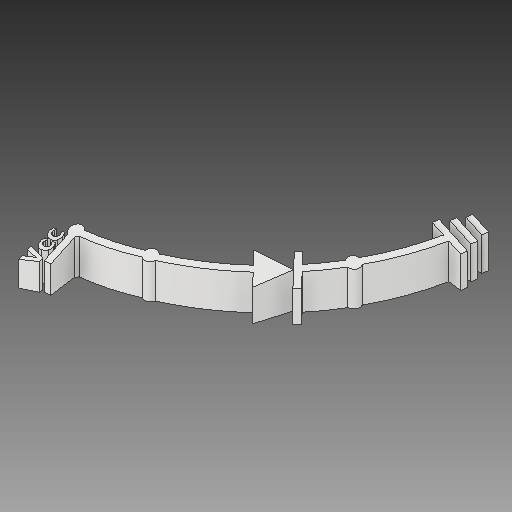
# Autodesk Inventor part: Mentor-Electrical text
Saved by Autodesk Inventor 2017 (Build 210142000, 142)
## iProperties
Created: 2016-02-20
Part Number: Mentor-Electrical text
Material: Generic
Document SubType Name: Modeling
Designer: RoksBot
Density: 1 g/cm^3
Appearance: White
Author: RoksBot
Autodesk Inventor part; units mm, degrees
ref_plane "YZ Plane" through (0, 0, 0) normal (1, 0, 0) x (0, 1, 0)
ref_plane "XZ Plane" through (0, 0, 0) normal (0, 1, 0) x (-1, 0, 0)
ref_plane "XY Plane" through (0, 0, 0) normal (0, 0, 1) x (1, 0, 0)
sketch "Sketch1" plane through (0, 0, 0) normal (0, 0, 1) x (1, 0, 0)
  line L0 (0, 0) -> (0, 8.6646) construction
  line L1 (20.9931, 1.27) -> (20.9931, 5.715)
  line L2 (20.9931, 5.715) -> (27.9781, 3.81)
  line L3 (27.9781, 3.81) -> (27.9781, 0)
  line L4 (27.9781, 0) -> (20.9931, 0)
  line L5 (20.9931, 1.27) -> (18.4531, 1.27)
  line L6 (18.4531, 1.27) -> (18.4531, 0)
  line L7 (18.4531, 0) -> (20.9931, 0)
  dimension "d0" = 20.9931
  dimension "d1" = 4.445
  dimension "d2" = 1.27
  dimension "d3" = 2.54
  dimension "d4" = 3.81
  dimension "d5" = 6.985
  constraints: 16 end point, 2 parallel, 2 perpendicular, 2 vertical, 1 horizontal, 1 horizontal alignment
  measures "d0" distance between parallel lines of L0 L1
  measures "d1" distance from line of L5 L1.end
  measures "d2" distance of L5.end L6.end
  measures "d3" distance between parallel lines of L1 L6
  measures "d4" distance of L2.end L3.end
  measures "d5" distance between parallel lines of L1 L3
revolve "Revolution1" add sketch "Sketch1" angle 360 about axis through (0, 0, 0) along (0, 1, 0)
sketch "Sketch2" plane through (0, 1.27, 0) normal (0, 1, 0) x (1, 0, 0)
  circle A0 centre (0, 0) radius 18.4531 projected
  circle A1 centre (0, 0) radius 20.9931 projected
  circle A2 centre (9.2057, -21.5899) radius 0.635
  arc A3 (9.6281, -21.1157) -> (15.5586, -17.2201) centre (0.0002, 0.0034) ccw
  arc A4 (9.8266, -21.7232) -> (15.9948, -17.6828) centre (0.0002, 0.0063) ccw
  line L0 (14.6057, -16.2094) -> (17.9425, -15.4197)
  line L1 (17.9425, -15.4197) -> (16.958, -18.7043)
  line L2 (16.958, -18.7043) -> (14.6057, -16.2094)
  line L3 (19.5807, -16.2316) -> (17.2284, -13.7366)
  line L4 (17.2284, -13.7366) -> (16.7663, -14.1722)
  line L5 (16.7663, -14.1722) -> (19.1186, -16.6672)
  line L6 (19.1186, -16.6672) -> (19.5807, -16.2316)
  line L7 (19.5807, -16.2316) -> (16.7663, -14.1722) construction
  line L8 (17.2284, -13.7366) -> (19.1186, -16.6672) construction
  arc A5 (18.0419, -14.5995) -> (19.8962, -11.96) centre (0.0423, 0.0164) ccw
  arc A6 (18.4961, -15.0813) -> (20.4645, -12.2797) centre (0.0089, 0.0003) ccw
  circle A7 centre (20.4475, -11.645) radius 0.635
  line L9 (22.5608, -1.3676) -> (24.4495, -1.6162)
  line L10 (24.4495, -1.6162) -> (24.3666, -2.2458)
  line L11 (24.3666, -2.2458) -> (22.4779, -1.9971)
  line L12 (22.4779, -1.9971) -> (22.5608, -1.3676)
  line L13 (22.5608, -1.3676) -> (24.3666, -2.2458) construction
  line L14 (24.4495, -1.6162) -> (22.4779, -1.9971) construction
  line L15 (22.0314, -3.2193) -> (24.5496, -3.5508)
  line L16 (24.5496, -3.5508) -> (24.6325, -2.9213)
  line L17 (24.6325, -2.9213) -> (22.1143, -2.5897)
  line L18 (22.1143, -2.5897) -> (22.0314, -3.2193)
  line L19 (22.0314, -3.2193) -> (24.6325, -2.9213) construction
  line L20 (24.5496, -3.5508) -> (22.1143, -2.5897) construction
  line L21 (21.3909, -4.4159) -> (24.7906, -4.8635)
  line L22 (24.7906, -4.8635) -> (24.8735, -4.2339)
  line L23 (24.8735, -4.2339) -> (21.4738, -3.7864)
  line L24 (21.4738, -3.7864) -> (21.3909, -4.4159)
  line L25 (21.3909, -4.4159) -> (24.8735, -4.2339) construction
  line L26 (24.7906, -4.8635) -> (21.4738, -3.7864) construction
  line L27 (0.0089, 0.0003) -> (33.281, -4.3801) construction
  arc A8 (20.9833, -11.3042) -> (23.3756, -4.6772) centre (0.0382, 0.0018) ccw
  arc A9 (20.3985, -11.0118) -> (22.7306, -4.5923) centre (0.0423, 0.0164) ccw
  line L28 (0.0423, 0.0164) -> (36.1387, 0.0164) construction
  circle A10 centre (0.0423, 0.0164) radius 23.4691 construction
  line L29 (0.0423, 0.0164) -> (5.4426, -41.0027) construction
  line L30 (0.0423, 0.0164) -> (0.0423, -40.9797) construction
  circle A11 centre (3.1056, -23.252) radius 0.635
  arc A12 (3.6155, -22.8735) -> (8.5745, -21.5207) centre (0.9957, -3.5037) ccw
  arc A13 (3.6826, -23.5172) -> (8.8414, -22.11) centre (1.5242, -5.4447) ccw
  line L31 (2.861, -23.8379) -> (3.2405, -26.7204)
  line L32 (3.2405, -26.7204) -> (3.87, -26.6375)
  line L33 (3.87, -26.6375) -> (3.4908, -23.7568)
  line L34 (1.3846, -26.2458) -> (2.9639, -26.5661)
  line L35 (2.9639, -26.5661) -> (3.016, -26.9616)
  line L36 (3.016, -26.9616) -> (1.5734, -27.6797)
  line L37 (1.5734, -27.6797) -> (1.5217, -27.2866)
  line L38 (1.5217, -27.2866) -> (2.5032, -26.8223)
  line L39 (2.5032, -26.8223) -> (1.4351, -26.6291)
  line L40 (1.4351, -26.6291) -> (1.3846, -26.2458)
  spline S0 degree 2 poles (2.8327, -25.3327) (2.8513, -25.4735) (2.811, -25.7167) (2.749, -25.8134) knots 0 0 0 1 2 2 2
  spline S1 degree 2 poles (2.749, -25.8134) (2.6854, -25.9077) (2.4739, -26.0327) (2.3221, -26.0527) knots 0 0 0 1 2 2 2
  spline S2 degree 2 poles (2.3221, -26.0527) (2.158, -26.0743) (1.9155, -26.0016) (1.8303, -25.9218) knots 0 0 0 1 2 2 2
  spline S3 degree 2 poles (1.8303, -25.9218) (1.7481, -25.8467) (1.6493, -25.6255) (1.6328, -25.5007) knots 0 0 0 1 2 2 2
  spline S4 degree 2 poles (1.6328, -25.5007) (1.6204, -25.4064) (1.6397, -25.212) (1.6748, -25.1102) knots 0 0 0 1 2 2 2
  line L41 (1.6748, -25.1102) -> (1.9785, -25.0702)
  line L42 (1.9785, -25.0702) -> (1.9845, -25.1155)
  spline S5 degree 2 poles (1.9845, -25.1155) (1.9666, -25.1403) (1.9256, -25.208) (1.9109, -25.2473) knots 0 0 0 1 2 2 2
  spline S6 degree 2 poles (1.9109, -25.2473) (1.894, -25.2894) (1.8774, -25.39) (1.8853, -25.45) knots 0 0 0 1 2 2 2
  spline S7 degree 2 poles (1.8853, -25.45) (1.9031, -25.5859) (2.1126, -25.7103) (2.2742, -25.689) knots 0 0 0 1 2 2 2
  spline S8 degree 2 poles (2.2742, -25.689) (2.4456, -25.6664) (2.5937, -25.485) (2.5763, -25.3528) knots 0 0 0 1 2 2 2
  spline S9 degree 2 poles (2.5763, -25.3528) (2.5674, -25.2854) (2.5236, -25.1891) (2.4967, -25.1552) knots 0 0 0 1 2 2 2
  spline S10 degree 2 poles (2.4967, -25.1552) (2.4712, -25.1225) (2.4179, -25.0772) (2.3971, -25.0612) knots 0 0 0 1 2 2 2
  line L43 (2.3971, -25.0612) -> (2.3911, -25.0159)
  line L44 (2.3911, -25.0159) -> (2.696, -24.9758)
  spline S11 degree 2 poles (2.696, -24.9758) (2.7135, -25.0046) (2.7583, -25.0797) (2.7748, -25.1199) knots 0 0 0 1 2 2 2
  spline S12 degree 2 poles (2.7748, -25.1199) (2.7963, -25.1694) (2.8229, -25.258) (2.8327, -25.3327) knots 0 0 0 1 2 2 2
  spline S13 degree 2 poles (2.6884, -24.2368) (2.707, -24.3777) (2.6667, -24.6209) (2.6047, -24.7175) knots 0 0 0 1 2 2 2
  spline S14 degree 2 poles (2.6047, -24.7175) (2.5412, -24.8118) (2.3297, -24.9368) (2.1778, -24.9568) knots 0 0 0 1 2 2 2
  spline S15 degree 2 poles (2.1778, -24.9568) (2.0138, -24.9784) (1.7712, -24.9057) (1.686, -24.826) knots 0 0 0 1 2 2 2
  spline S16 degree 2 poles (1.686, -24.826) (1.6039, -24.7508) (1.505, -24.5297) (1.4885, -24.4048) knots 0 0 0 1 2 2 2
  spline S17 degree 2 poles (1.4885, -24.4048) (1.4761, -24.3105) (1.4954, -24.1161) (1.5306, -24.0143) knots 0 0 0 1 2 2 2
  line L45 (1.5306, -24.0143) -> (1.8342, -23.9744)
  line L46 (1.8342, -23.9744) -> (1.8402, -24.0197)
  spline S18 degree 2 poles (1.8402, -24.0197) (1.8223, -24.0444) (1.7814, -24.1121) (1.7666, -24.1514) knots 0 0 0 1 2 2 2
  spline S19 degree 2 poles (1.7666, -24.1514) (1.7497, -24.1935) (1.7331, -24.2941) (1.741, -24.3541) knots 0 0 0 1 2 2 2
  spline S20 degree 2 poles (1.741, -24.3541) (1.7589, -24.49) (1.9683, -24.6144) (2.13, -24.5931) knots 0 0 0 1 2 2 2
  spline S21 degree 2 poles (2.13, -24.5931) (2.3014, -24.5706) (2.4494, -24.3891) (2.432, -24.2569) knots 0 0 0 1 2 2 2
  spline S22 degree 2 poles (2.432, -24.2569) (2.4231, -24.1896) (2.3793, -24.0932) (2.3524, -24.0594) knots 0 0 0 1 2 2 2
  spline S23 degree 2 poles (2.3524, -24.0594) (2.3269, -24.0266) (2.2736, -23.9813) (2.2528, -23.9653) knots 0 0 0 1 2 2 2
  line L47 (2.2528, -23.9653) -> (2.2469, -23.92)
  line L48 (2.2469, -23.92) -> (2.5518, -23.8799)
  spline S24 degree 2 poles (2.5518, -23.8799) (2.5693, -23.9087) (2.614, -23.9838) (2.6305, -24.024) knots 0 0 0 1 2 2 2
  spline S25 degree 2 poles (2.6305, -24.024) (2.652, -24.0735) (2.6786, -24.1622) (2.6884, -24.2368) knots 0 0 0 1 2 2 2
  point P0 (16.502, -16.7778)
  point P1 (15.7818, -17.4569)
  point P2 (18.1735, -15.2019)
  point P3 (23.4637, -1.8067)
  point P4 (23.332, -3.0703)
  point P5 (23.1322, -4.3249)
  point P6 (23.332, -3.0703)
  dimension "d48" = 1.27
  dimension "d50" = 0.635
  dimension "d52" = 7.62
  dimension "d53" = 3.429
  dimension "d54" = 0.635
  dimension "d55" = 3.429
  dimension "d56" = 1.27
  dimension "d57" = 0.635
  dimension "d59" = 3.81
  dimension "d60" = 3.429
  dimension "d61" = 2.54
  dimension "d62" = 1.905
  dimension "d63" = 0.635
  dimension "d64" = 0.635
  dimension "d65" = 0.635
  dimension "d67" = 0.635
  dimension "d74" = 7.5
  dimension "d75" = 0.3175
  dimension "d77" = 7.5
  dimension "d78" = 0.635
  constraints: 68 end point, 30 point on circle, 16 parallel, 12 centre point, 11 midpoint, 8 point on line, 5 perpendicular, 1 coincident, 1 concentric, 1 equal radius, 1 horizontal, 1 vertical, 8 other
  measures "d48" diameter of A2
  measures "d52" distance from line of L2 A2.centre
  measures "d53" distance of L1.end L0.start
  measures "d54" distance between parallel lines of L5 L3
  measures "d55" distance of L4.end L5.end
  measures "d56" diameter of A7
  measures "d59" distance of A5.start A7.centre
  measures "d60" distance of L21.start L21.end
  measures "d61" distance of L15.start L15.end
  measures "d62" distance of L10.end L11.end
  measures "d63" distance of L9.end L10.end
  measures "d64" distance between parallel lines of L23 L15
  measures "d65" distance between parallel lines of L17 L11
  measures "d74" angle of L28 L27
  measures "d75" radial gap between concentric circles of A9 A10
  measures "d77" angle of L30 L29
  measures "d78" distance of L31.end L32.end
extrude "Extrusion1" cut sketch "Sketch2" along normal through all contours A2 | A2 A3 L2 A4 | L5 L4 L3 L6 | A2 A13 A11 A12 | L2 L0 L1 | A11 | A11 L33 L32 L31 | A5 A7 A6 L3 | A7 | A9 L21 A8 A7 | L21 L24 L23 L22 | L9 L10 L11 L12 | L18 L17 L16 L15 | L34 L35 L36 L37 L38 L39 L40 | S0 S1 S2 S3 S4 L41 L42 S5 S6 S7 S8 S9 S10 L43 L44 S11 S12 | S13 S14 S15 S16 S17 L45 L46 S18 S19 S20 S21 S22 S23 L47 L48 S24 S25 keep common part
sketch "Sketch4" plane through (0, 1.27, 0) normal (0, 1, 0) x (1, 0, 0)
  line L0 (0, 0) -> (37.9646, 0)
  line L1 (37.9646, 0) -> (37.9646, -33.7381)
  line L2 (37.9646, -33.7381) -> (0, -33.7381)
  line L3 (0, -33.7381) -> (0, 0)
  constraints: 8 end point, 2 parallel, 1 horizontal, 1 perpendicular
extrude "Extrusion3" cut sketch "Sketch4" along normal through all both and the other way through all keep common part
equation "\"d48\" = d35"
equation "\"d52\" = d49"
equation "\"d53\" = d39"
equation "\"d54\" = d42"
equation "\"d55\" = d53"
equation "\"d56\" = d48"
equation "\"d59\" = d34"
equation "\"d65\" = d64"
equation "\"d26\" = d18"
equation "\"d35\" = d26"
equation "\"d39\" = d29"
equation "\"d40\" = d36"
equation "\"d42\" = d31"
equation "\"d49\" = d40"
equation "\"d34\" = 3.81"
equation "\"d18\" = 1.27"
equation "\"d29\" = 3.429"
equation "\"d36\" = 7.62"
equation "\"d31\" = 0.635"
body "Solid1"
